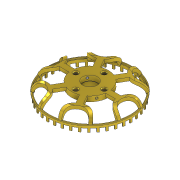
# Autodesk Inventor part: outrunner
Saved by Autodesk Inventor 2020 (Build 240168000, 168)
## iProperties
Created: 2020-05-19
Part Number: outrunner
Material: Generic
Document SubType Name: Modeling
Designer: Kostic
Density: 1 g/cm^3
Appearance: Aluminum - Polished
Author: Kostic
Autodesk Inventor part; units mm, degrees
ref_plane "YZ Plane" through (0, 0, 0) normal (1, 0, 0) x (0, 1, 0)
ref_plane "XZ Plane" through (0, 0, 0) normal (0, 1, 0) x (-1, 0, 0)
sketch "Sketch1" plane through (0, 0, 0) normal (0, 0, 1) x (1, 0, 0)
  line L0 (0, 0) -> (0, 71.3243) construction
  line L1 (0, 6.5) -> (34.5, 6.5)
  line L2 (34.5, 6.5) -> (34.5, 10)
  line L3 (34.5, 10) -> (0, 10)
  line L4 (0, 10) -> (0, 6.5)
  line L5 (45.9, 0) -> (43.9, 0)
  line L6 (43.9, 0) -> (43.9, 1)
  line L7 (43.9, 1) -> (45.9, 1)
  line L8 (45.9, 1) -> (45.9, 0)
  line L9 (45.9, 0) -> (43.9, 0)
  line L10 (43.9, 0) -> (43.9, -7)
  line L11 (43.9, -7) -> (44.9, -7)
  line L12 (44.9, -7) -> (44.9, 0)
  arc A0 (45.9, 1) -> (34.5, 10) centre (34.5, -1.72) ccw
  line L13 (0, 0) -> (87.4333, 0) construction
  arc A1 (43.9, -1.5) -> (34.5, 6.5) centre (34.5, -3.0225) ccw
  line L14 (0, 5.0307) -> (8, 5.0307)
  line L15 (8, 5.0307) -> (8, 19.046)
  line L16 (8, 19.046) -> (0, 19.046)
  line L17 (0, 19.046) -> (0, 5.0307)
  point P0 (8, 10)
  point P1 (8, 6.5)
  point P2 (44.9, 0)
  dimension "d0" = 7
  dimension "d1" = 43.9
  dimension "d2" = 44.9
  dimension "d3" = 45.9
  dimension "d4" = 1
  dimension "d6" = 3.5
  dimension "d7" = 34.5
  dimension "d8" = 10
  dimension "d9" = 0
  dimension "d10" = 1.5
  dimension "d11" = 8
  constraints: 36 end point, 8 parallel, 5 horizontal, 4 perpendicular, 4 point on circle, 3 point on line, 2 centre point, 2 tangent, 1 collinear, 1 vertical
  measures "d0" distance between parallel lines of L5 L11
  measures "d1" distance between parallel lines of L0 L10
  measures "d2" distance between parallel lines of L0 L12
  measures "d3" distance between parallel lines of L0 L8
  measures "d4" distance between parallel lines of L5 L7
  measures "d6" distance between parallel lines of L1 L3
  measures "d7" distance between parallel lines of L4 L2
  measures "d8" distance from line of L0.start L3
  measures "d9" distance between parallel lines of L10 L6
  measures "d10" distance from line of A1.start L13
  measures "d11" distance of L16.end L15.end
revolve "Revolution1" add sketch "Sketch1" angle 360 about axis through (0, 0, 0) along (0, 1, 0) contours L15 L3 L2 L1 | L2 A0 L7 L6 L10 A1 | L10 L5 L12 L11 | L8 L5 L6 L7
sketch "Sketch2" plane through (0, 10, 0) normal (0, 1, 0) x (1, 0, 0)
  line L0 (0, 0) -> (25.8201, 44.7218) construction
  line L1 (0, 0) -> (51.6403, 0) construction
  line L2 (0, 0) -> (10.0393, 44.7886) construction
  line L3 (0, 0) -> (33.7684, 31.0886) construction
  circle A0 centre (0, 0) radius 45.9 projected
  line L4 (0, 0) -> (13.0512, 44.0054) construction
  line L5 (0, 0) -> (31.5842, 33.3054) construction
  arc A1 (13.0512, 44.0054) -> (31.5842, 33.3054) centre (22.3501, 38.7115) ccw
  line L6 (0, 0) -> (17, 29.4449) construction
  line L7 (0, 0) -> (15.25, 26.4138) construction
  arc A2 (10.0393, 44.7886) -> (33.7684, 31.0886) centre (22.1029, 38.2833) ccw
  circle A3 centre (0, 0) radius 8 projected
  circle A4 centre (0, 0) radius 20.15
  line L8 (6.2442, 16.8152) -> (13.6297, 29.6074)
  line L9 (13.6297, 29.6074) -> (18.8259, 26.6074)
  line L10 (18.8259, 26.6074) -> (11.4403, 13.8152)
  line L11 (11.4403, 13.8152) -> (6.2442, 16.8152)
  point P0 (7.3646, 18.7559)
  point P1 (12.5608, 15.7559)
  point P2 (18.0143, 25.2016)
  point P3 (12.8181, 28.2016)
  dimension "d13" = 60
  dimension "d14" = 27.4
  dimension "d15" = 21.4
  dimension "d16" = 91.8
  dimension "d18" = 34
  dimension "d19" = 30.5
  dimension "d20" = 40.3
  dimension "d21" = 6
  dimension "d22" = 3
  constraints: 24 end point, 10 point on circle, 3 centre point, 3 parallel, 2 point on line, 1 coincident, 1 equal length, 1 horizontal, 1 perpendicular, 2 other
  measures "d13" angle of L1 L0
  measures "d14" distance of L3.end L2.end
  measures "d15" distance of L5.end L4.end
  measures "d16" diameter of A0
  measures "d18" distance of L4.start L6.end
  measures "d19" distance of L4.start L7.end
  measures "d20" diameter of A4
  measures "d21" distance of L8.end L9.end
  measures "d22" distance between parallel lines of L8 L7
extrude "Extrusion1" cut sketch "Sketch2" against normal blind 20 contours A2 L10 L9 L8 A0 A1 | L10 A4 L8 A2 | A2 L8 L9 L10 | L10 L11 L8 A4 | A4 L8 L11 L10 keep common part
pattern_circular "Circular Pattern1" count 6 over 360 about axis through (0, 8.25, 0) along (0, -1, 0)
sketch "Sketch3" plane through (0, -7, 0) normal (0, -1, 0) x (0.7176936, 0, -0.696359)
  circle A0 centre (0, 0) radius 44.9
  arc A1 (-43.8725, 1.5549) -> (-43.8725, -1.5549) centre (0, 0) ccw projected
  circle A2 centre (0, 0) radius 43.9
  point P0 (-43.8725, 1.5549)
  constraints: 2 coincident, 1 centre point, 3 other
extrude "Extrusion2" add sketch "Sketch3" against normal up to surface (7 mm away)
sketch "Sketch4" plane through (0, 0, 0) normal (0, -1, 0) x (0.7123115, 0, 0.7018635)
  circle A0 centre (0, 0) radius 45.9
  circle A1 centre (0, 0) radius 44.9
  constraints: 2 centre point, 2 coincident
extrude "Extrusion3" add sketch "Sketch4" against normal blind 1
sketch "Sketch5" plane through (0, -7, 0) normal (0, -1, 0) x (1, 0, 0)
  line L0 (-47.1897, -2.5) -> (-47.1897, 2.5)
  line L1 (-47.1897, 2.5) -> (-38.9034, 2.5)
  line L2 (-38.9034, 2.5) -> (-38.9034, -2.5)
  line L3 (-38.9034, -2.5) -> (-47.1897, -2.5)
  point P0 (0, 0)
  dimension "d32" = 5
  dimension "d33" = 2.5
  constraints: 8 end point, 2 parallel, 1 perpendicular, 1 vertical
  measures "d32" distance of L0.start L0.end
  measures "d33" distance from line of point (0, 0) L3
extrude "Extrusion4" cut sketch "Sketch5" against normal blind 4
sketch "Sketch7" plane through (0, 6.5, 0) normal (0, -1, 0) x (1, 0, 0)
  circle A0 centre (0, 0) radius 20.15
  circle A1 centre (0, 0) radius 8
  constraints: 2 centre point, 2 coincident
extrude "Extrusion5" add sketch "Sketch7" along normal blind 2
pattern_circular "Circular Pattern2" count 39 over 360 about axis through (0, -3.5, 0) along (0, -1, 0) of "Extrusion4"
sketch "Sketch6" plane through (0, 10, 0) normal (0, 1, 0) x (1, 0, 0)
  circle A0 centre (-15.5, 0) radius 2.5
  circle A1 centre (0, -15.5) radius 2.5
  circle A2 centre (15.5, 0) radius 2.5
  circle A3 centre (0, 15.5) radius 2.5
  point P0 (0, 0)
  dimension "d39" = 5
  dimension "d40" = 15.5
  dimension "d43" = 360
  constraints: 4 centre point, 9 other
  measures "d39" diameter of A0
  measures "d40" distance of point (0, 0) A0.centre
hole "Hole1" at (-15.5, 10, 0) at (0, 10, -15.5) at (15.5, 10, 0) at (0, 10, 15.5) direction (0, -1, 0) diameter 4.134 end through all countersink diameter 6 countersink angle 90 thread size "M5x0.8" class "6H" standard "ISO Metric profile"
sketch "Sketch8" plane through (0, 4.5, 0) normal (0, -1, 0) x (1, 0, 0)
  circle A0 centre (0, 0) radius 7.5
  circle A1 centre (0, 0) radius 10.5
  circle A2 centre (0, 0) radius 8 projected
  dimension "d54" = 21
  dimension "d60" = 15
  constraints: 2 centre point, 2 coincident
  measures "d54" diameter of A1
  measures "d60" diameter of A0
extrude "Extrusion6" add sketch "Sketch8" along normal blind 7.5 contours A1 | A2
chamfer "Chamfer2" distance 2 distance2 1.5 1 edges at (-10.5, -3, 0) measured on face at (-10, -3, 0)
ref_plane "Work Plane2" through (-30.8324, 10, -3) normal (0.8660254, 0, 0.5) x (0, -1, 0)
sketch "Sketch10" plane through (-30.8324, 10, -3) normal (0.8660254, 0, 0.5) x (0, -1, 0)
  circle A0 centre (2.5, 12.8181) radius 1.5
  line L0 (0, 5.4535) -> (0, 20.1827) projected
  point P0 (10, 12.8181)
  dimension "d64" = 3
  dimension "d65" = 2.5
  dimension "d66" = 0
  constraints: 1 centre point
  measures "d64" diameter of A0
  measures "d65" distance from line of L0 A0.centre
  measures "d66" vertical distance of A0.centre point (10, 12.818)
hole "Hole2" at (-24.4233, 7.5, -14.1008) direction (0.8660254, 0, 0.5) diameter 2.459 end through all thread size "M3x0.5" class "6H" standard "ISO Metric profile"
equation "\"d33\" = 0.5 * d32"
body "Solid1"
